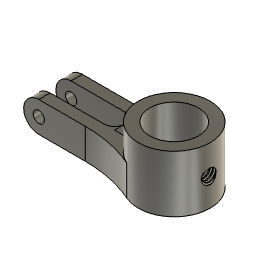
Mount for Half Inch Rod Perpendicular v8 (Autodesk Fusion 360 design; units mm, degrees)
Autodesk Fusion 360 part; units mm, degrees
note: some values were not read from the file. Chosen so that the rebuilt part matches the saved one: which bodies a step acts on; which face or edge a step refers to; where a thread starts. Set by a fixed rule: which sketch regions a step uses.
sketch "Sketch1" plane through (0, 0, 0) normal (0, 0, 1) x (1, 0, 0)
  circle A0 centre (0, 0) radius 6.425
  circle A1 centre (0, 0) radius 9.5
  dimension "d28" = 12.85
  dimension "d29" = 19
  constraint coincident A0.centre A1.centre
  measures "d28" diameter of A0
  measures "d29" diameter of A1
sketch "Sketch2" plane through (0, 0, 0) normal (0, 0, 1) x (1, 0, 0)
  line L0 (0, 0) -> (-20, 0)
  constraint coincident L0.start origin
  constraint horizontal L0
sketch "Sketch3" plane through (0, 0, 0) normal (0, 0, 1) x (1, 0, 0)
  line L0 (0, 0) -> (-9.5, 0)
  line L1 (-9.5, 0) -> (-19.5, 0)
  circle A0 centre (-19.5, 0) radius 1.5025
  arc A1 (-19.5, 4) -> (-19.5, -4) centre (-19.5, 0) ccw
  line L2 (-19.5, 4) -> (-10, 4)
  line L3 (-19.5, -4) -> (-10, -4)
  line L4 (-10, -4) -> (-6.25, -7.15)
  line L5 (-6.25, 7.15) -> (-10, 4)
  line L6 (-6.25, -7.15) -> (-8, 0)
  line L7 (-8, 0) -> (-6.25, 7.15)
  dimension "d30" = 9.5
  dimension "d31" = 10
  dimension "d32" = 3.005
  dimension "d33" = 4
  dimension "d34" = 14.3
  constraint coincident L0.start origin
  constraint horizontal L0
  constraint parallel L0 L1
  constraint coincident L1.end A0.centre
  constraint tangent A1 L2
  constraint horizontal L2
  constraint tangent A1 L3
  constraint horizontal L3
  constraint coincident L0 L6.end
  measures "d30" distance of L0.start L0.end
  measures "d31" distance of L0.end L1.end
  measures "d32" diameter of A0
  measures "d33" radius of A1
  measures "d34" distance of L4.end L5.start
extrude "Extrude1" add sketch "Sketch1" along normal mid plane 15 makes body 1
hole "Hole1" at (9.5, 0, -0.0147) direction (-1, 0, 0) diameter 3.416 depth 5 tip angle 180 bodies 1
thread "Thread1" "ANSI Unified Screw Threads 0.164(#8) 8-32 UNC 2B"
thread "Thread2" "ANSI Unified Screw Threads 0.164(#8) 8-32 UNC 2B" major diameter 4.1656 minor diameter 3.4163 pitch 0.7937 angle 60 modelled right hand crest width 0.2341 on face at (8.4537, 0.5924, -1.6167) crest through (9.8969, 0, -1.7229) on bodies 1
sketch "Sketch5" plane through (0, 0, 0) normal (0, 1, 0) x (1, 0, 0)
  line L0 (-9.5, 0) -> (-25, 0)
  arc A0 (-25, 4) -> (-25, -4) centre (-25, 0) ccw
  line L1 (-25, -4) -> (-9.5, -4)
  line L2 (-9.5, -4) -> (-9.5, 4)
  line L3 (-9.5, 4) -> (-25, 4)
  circle A1 centre (-25, 0) radius 1.503
  line L4 (-21.873, 1.8054) -> (-25, 3.6107)
  line L5 (-25, 3.6107) -> (-28.127, 1.8054)
  line L6 (-28.127, 1.8054) -> (-28.127, -1.8054)
  line L7 (-28.127, -1.8054) -> (-25, -3.6107)
  line L8 (-25, -3.6107) -> (-21.873, -1.8054)
  line L9 (-21.873, -1.8054) -> (-21.873, 1.8054)
  line L10 (-9.5, -4) -> (-6.4645, -4)
  line L11 (-6.4645, -4) -> (-6.4645, 4)
  line L12 (-6.4645, 4) -> (-9.5, 4)
  point P0 (-25, 0)
  dimension "d36" = 3.006
  dimension "d37" = 3.127
  constraint horizontal L0
  constraint coincident P0 L0.end
  constraint tangent A0 L1
  constraint horizontal L1
  constraint perpendicular L1 L2
  constraint tangent A0 L3
  constraint concentric A0 A1
  constraint perpendicular L2 L10
  constraint perpendicular L10 L11
  constraint perpendicular L2 L12
  measures "d36" diameter of A1
  measures "d37" distance of P0 L9
extrude "Extrude7" add sketch "Sketch5" along normal blind 2.5 from surface at 2.753 separate body contours A0 L1 L2 L3 | L2 L10 L11 L12 | L4 L5 L6 L7 L8 L9 makes body 2
extrude "Extrude8" add sketch "Sketch5" against normal blind 2.5 from surface at -2.753 separate body contours A0 L1 L2 L3 | L2 L10 L11 L12 | L4 L5 L6 L7 L8 L9 makes body 3
extrude "Extrude9" cut sketch "Sketch5" along normal blind 4.5 from surface at 5 contours L4 L5 L6 L7 L8 L9 bodies 2
extrude "Extrude10" add 1 faces at (-11.6006, 5.253, -0.6018) along direction (0, 1, 0) blind 0.5 on bodies 2 bodies 2
move_body "Move1" bodies 2 to x (1, 0, 0) y (0, 1, 0) z (0, 0, 1) at (0, 0, -3.5)
move_body "Move2" bodies 3 to x (1, 0, 0) y (0, 1, 0) z (0, 0, 1) at (0, 0, -3.5)
combine "Combine1" operation add target body 1 tool bodies 2 3
sketch "Sketch6" plane through (0, 0, 0) normal (0, 0, 1) x (1, 0, 0)
  line L0 (-15, -20) -> (-15, 10)
  constraint vertical L0
split "Split1" by curves path "Sketch6" along L0 bodies 1 makes body 4 at (-17.8323, -2.753, -3.5) makes body 5 at (8.8733, -3.3932, 0.0075)
move_body "Move3" bodies 4 to x (1, 0, 0) y (0, 1, 0) z (0, 0, 1) at (-5, 0, 0)
move_body "Move4" bodies 1 to x (1, 0, 0) y (0, 1, 0) z (0, 0, 1) at (-5, 0, 0)
extrude "Extrude11" add 2 faces at (-15, 3.753, -4.8333) (-15, -4.4197, -4.8333) along direction (-1, 0, 0) blind 5 on bodies 5 bodies 5 1 4
extrude "Extrude12" add 1 faces at (-19.3052, -5.253, -2.1667) along direction (0, -1, 0) blind 0.5 on bodies 5 bodies 5
extrude "Extrude13" add 1 faces at (-7.9156, -5.5863, -2.1667) along direction (1, 0, 0) blind 0.5 on bodies 5 bodies 5
sketch "Sketch7" plane through (0, -2.753, 0) normal (0, 1, 0) x (-1, 0, 0)
  circle A0 centre (30, -3.5) radius 1.503
  line L0 (30, 0.5) -> (9.0924, 0.5)
  line L1 (9.0924, 0.5) -> (9.0924, -7.5)
  line L2 (9.0924, -7.5) -> (30, -7.5)
  arc A1 (30, -7.5) -> (30, 0.5) centre (30, -3.5) ccw
  line L3 (13, 0) -> (13, 0.5)
  line L4 (13, 0.5) -> (13, -7.5)
  line L5 (13, -7.5) -> (8, -7.5)
  line L6 (8, -7.5) -> (8, 0.5)
  line L7 (8, 0.5) -> (13, 0.5)
  constraint coincident L0 L3.end
  constraint perpendicular L0 L3
  constraint coincident L2 L4.end
  constraint perpendicular L2 L4
  constraint perpendicular L1 L5
  constraint perpendicular L5 L6
extrude "Extrude14" add sketch "Sketch7" along normal blind 8 contours L0 L1 L2 L3 L4 L5 L7 bodies 5
fillet "Fillet1" radius 2.75 2 edges at (-13, -2.753, -3.5) (-13, 2.753, -3.5) on bodies 5
fillet "Fillet2" radius 34.5 2 edges at (-7.56, 5.753, -3.5) (-7.56, -5.753, -3.5) on bodies 5
named bodies: "Sleeve Camera Mount 2"
